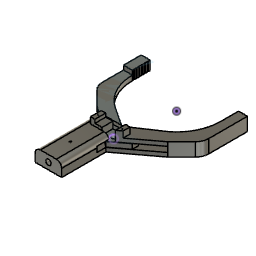
klo (Autodesk Fusion 360 design; units mm, degrees)
Autodesk Fusion 360 part; units mm, degrees
sketch "Sketch1" plane through (0, 0, 0) normal (0, 0, 1) x (1, 0, 0)
  circle A0 centre (0, 0) radius 50
  circle A1 centre (0, 0) radius 40 construction
  line L0 (45.8258, 20) -> (60, 20)
  line L1 (60, 20) -> (60, -30)
  line L2 (0, 0) -> (0, -40)
  line L3 (0, -60) -> (25.3846, -43.0769)
  line L4 (0, -80) -> (40, -50)
  line L5 (40, -50) -> (60, -30)
  line L6 (0, -80) -> (-30, -80)
  line L7 (-30, -60) -> (-30, -80)
  line L8 (0, -60) -> (-30, -60)
  dimension "d1" = 100
  constraint coincident A0.centre A1.centre
  constraint concentric A0 A1
  constraint perpendicular L0 L1
  constraint coincident A1 L2.end
  constraint coincident A0 L0.start
  constraint coincident A0 L3.end
  constraint horizontal L6
  constraint perpendicular L6 L7
  constraint perpendicular L7 L8
  measures "d1" diameter of A0
extrude "Extrude1" add sketch "Sketch1" along normal blind 15 contours A0 L0 L1 L3 L4 L5 L6 L7 L8 makes body 1
sketch "Sketch2" plane through (0, 0, 15) normal (0, 0, 1) x (-1, 0, 0)
  line L0 (-25.3846, 43.0769) -> (0, 60)
  line L1 (0, 60) -> (30, 60)
  line L2 (30, 60) -> (30, 80)
  line L3 (30, 80) -> (0, 80)
  line L4 (0, 80) -> (-40, 50)
  line L5 (-40, 50) -> (-60, 30)
  line L6 (-60, 30) -> (-60, -20)
  line L7 (-60, -20) -> (-45.8258, -20)
  arc A0 (-25.3846, 43.0769) -> (-45.8258, -20) centre (0, 0) ccw
  circle A1 centre (0, 70) radius 5
  dimension "d4" = 10
  measures "d4" diameter of A1
ref_plane "WorkPlane6" through (0, 0, 7.5) normal (0, 0, 1) x (1, 0, 0)
sketch "Sketch4" plane through (0, 0, 7.5) normal (0, 0, 1) x (1, 0, 0)
  circle A0 centre (0, 0) radius 50
  line L0 (60, 20) -> (45.8258, 20)
  line L1 (60, 20) -> (60, -30)
  line L2 (0, -80) -> (-30, -80)
  line L3 (-30, -80) -> (-30, -60)
  line L4 (-30, -60) -> (0, -60)
  line L5 (0, -60) -> (27.6385, -41.6667)
  line L6 (0, -80) -> (40, -50)
  line L7 (40, -50) -> (60, -30)
  line L8 (0, 2.5) -> (0, 20)
  line L9 (30, -60) -> (0, -60)
  line L10 (-60, 20) -> (-60, -30)
  circle A1 centre (0, 0) radius 50
  line L11 (0, -80) -> (30, -80)
  line L12 (-40, -50) -> (-60, -30)
  line L13 (0, -60) -> (-27.6385, -41.6667)
  line L14 (-60, 20) -> (-45.8258, 20)
  line L15 (0, -80) -> (-40, -50)
  line L16 (30, -80) -> (30, -60)
  constraint coincident A0.centre A1.centre
  constraint coincident A0 L0.end
  constraint horizontal L0
  constraint perpendicular L0 L1
  constraint perpendicular L1 L2
  constraint perpendicular L0 L3
  constraint perpendicular L3 L4
  constraint coincident A0 L5.end
  constraint tangent A0 L5
  constraint symmetric A0.centre L8 A1.centre
  constraint symmetric A0 L8 A1
  constraint symmetric L0.start L8 L10.start
  constraint symmetric L0.end L8 L14.end
  constraint symmetric L1.end L8 L10.end
  constraint symmetric L2.start L8 L6.start
  constraint symmetric L2.end L8 L11.end
  constraint symmetric L3.end L8 L9.start
  constraint symmetric L4.end L8 L5.start
  constraint symmetric L5.end L8 L13.end
  constraint symmetric L6.end L8 L12.start
extrude "Extrude1'" add sketch "Sketch4" along normal blind 2.75 and the other way blind 2.75 separate body contours A0 L4 L10 A1 L12 L13 L14 L15 | L4 L6 L9 L15 | L6 L9 L11 L16 makes body 2 in component "Component"
ref_plane "WorkPlane1" through (20, -65, 7.5) normal (0.6, -0.8, 0) x (0.8, 0.6, 0) in component "Component"
sketch "Sketch1 (2)" plane through (20, -65, 10) normal (0.6, -0.8, 0) x (0.8, 0.6, 0) in component "Component"
  line L0 (-25, 5) -> (11, 5)
  line L1 (11, 5) -> (11, -5)
  line L2 (11, -5) -> (-25, -5)
  line L3 (-25, -5) -> (-25, 5)
  constraint horizontal L0
  constraint perpendicular L0 L1
  constraint perpendicular L1 L2
extrude "Extrude2" cut sketch "Sketch1 (2)" along normal blind 22 bodies 2 in component "Component"
sketch "Sketch5" plane through (0, 0, 7.5) normal (0, 0, 1) x (1, 0, 0)
  line L0 (0, -60) -> (-30, -60)
  line L1 (-30, -60) -> (-30, -80)
  line L2 (-30, -80) -> (0, -80)
  line L3 (0, -80) -> (40, -50)
  line L4 (40, -50) -> (30, -40)
  line L5 (30, -40) -> (0, -60)
  constraint horizontal L0
  constraint perpendicular L0 L1
  constraint perpendicular L1 L2
extrude "Extrude3" cut sketch "Sketch5" along normal blind 3 and the other way blind 3 bodies 1
extrude "Extrude4" cut sketch "Sketch2" against normal blind 4.5 contours A1 bodies 1
extrude "Extrude3'" [no effect] in component "Component"
sketch "Sketch13" plane through (0, 0, 10.25) normal (0, 0, 1) x (-1, 0, 0)
  line L0 (0, 80) -> (-26.6667, 60)
  line L1 (-26.6667, 60) -> (0, 60)
  line L2 (0, 60) -> (27.6385, 41.6667)
  arc A0 (45.8258, -20) -> (27.6385, 41.6667) centre (0, 0) ccw
  line L3 (45.8258, -20) -> (60, -20)
  line L4 (60, -20) -> (60, 30)
  line L5 (60, 30) -> (40, 50)
  line L6 (40, 50) -> (0, 80)
  line L7 (0, 70) -> (0.2128, 70)
  line L8 (0, 66) -> (0, 74) construction
  circle A1 centre (0, 70) radius 3.5
  line L9 (-2.9142, 68.0616) -> (-13.1179, 63.9525)
  circle A2 centre (-13.1179, 63.9525) radius 2
  line L10 (-1.7875, 73.0091) -> (-14.1393, 65.672)
  line L11 (1.1273, 66.6865) -> (-12.4737, 62.0591)
  dimension "d58" = 7
  dimension "d61" = 11
  dimension "d62" = 4
  constraint vertical L8
  constraint coincident A1 L9.start
  constraint coincident L9.end A2.centre
  constraint coincident A1 L10.start
  constraint coincident A2 L10.end
  constraint tangent A2 L10
  constraint coincident A1 L11.start
  constraint coincident A2 L11.end
  constraint tangent A2 L11
  constraint tangent A1 L11
  constraint tangent A1 L10
  measures "d58" diameter of A1
  measures "d61" distance of L9.start L9.end
  measures "d62" diameter of A2
sketch "Sketch14" plane through (0, 0, 0) normal (0, 0, -1) x (1, 0, 0)
  line L0 (0, 60) -> (25.3846, 43.0769)
  arc A0 (45.8258, -20) -> (25.3846, 43.0769) centre (0, 0) ccw
  line L1 (45.8258, -20) -> (60, -20)
  line L2 (60, -20) -> (60, 30)
  line L3 (60, 30) -> (40, 50)
  line L4 (40, 50) -> (0, 80)
  line L5 (0, 80) -> (-30, 80)
  line L6 (-30, 80) -> (-30, 60)
  line L7 (-30, 60) -> (0, 60)
  circle A1 centre (0, 70) radius 5
sketch "Sketch6" plane through (0, -80, 0) normal (0, -1, 0) x (1, 0, 0)
  line L0 (0, 10.5) -> (0, 15)
  line L1 (-30, 15) -> (-30, 10.5)
  line L2 (-30, 15) -> (0, 15)
  line L3 (0, 15) -> (0, 0)
  line L4 (0, 0) -> (-30, 0)
  line L5 (-30, 0) -> (-30, 15)
  line L6 (-30, 10.5) -> (0, 10.5)
  line L7 (0, 15) -> (-30, 15)
  constraint horizontal L2
  constraint vertical L3
  constraint horizontal L4
  constraint vertical L5
  constraint coincident L3.end L4.start
  constraint coincident L1.start L2.start
sketch "Sketch7" plane through (0, 0, 10.25) normal (0, 0, 1) x (-1, 0, 0)
  line L0 (0, 80) -> (-26.6667, 60)
  line L1 (-26.6667, 60) -> (0, 60)
  line L2 (0, 60) -> (27.6385, 41.6667)
  arc A0 (45.8258, -20) -> (27.6385, 41.6667) centre (0, 0) ccw
  line L3 (45.8258, -20) -> (60, -20)
  line L4 (60, -20) -> (60, 30)
  line L5 (60, 30) -> (40, 50)
  line L6 (40, 50) -> (0, 80)
  line L7 (-10, 60) -> (-10, 72.5)
  line L8 (-26.6667, 60) -> (-10, 60)
  line L9 (-10, 72.5) -> (-26.6667, 60)
  constraint coincident L1 L7.start
  constraint coincident L0 L7.end
  constraint perpendicular L1 L7
  constraint coincident L0.end L1.start
  constraint perpendicular L7 L8
  constraint parallel L0 L9
extrude "Extrude4'" cut sketch "Sketch7" against normal blind 30 contours L0 L1 L7 L8 L9 bodies 2 in component "Component"
sketch "Sketch8" plane through (0, -80, 0) normal (0, -1, 0) x (1, 0, 0)
  line L0 (0, 10.5) -> (0, 15)
  line L1 (-30, 15) -> (-30, 10.5)
  line L2 (-30, 15) -> (0, 15)
  line L3 (0, 15) -> (0, 10.5)
  line L4 (0, 10.5) -> (-30, 10.5)
  line L5 (-30, 10.5) -> (-30, 15)
  line L6 (-30, 4.5) -> (0, 4.5)
  line L7 (0, 4.5) -> (0, 0)
  line L8 (0, 0) -> (-30, 0)
  line L9 (-30, 0) -> (-30, 4.5)
  line L10 (-30, 10.5) -> (0, 10.5)
  line L11 (0, 15) -> (-30, 15)
  constraint horizontal L2
  constraint vertical L3
  constraint horizontal L4
  constraint vertical L5
  constraint coincident L0.start L3.end
  constraint coincident L1.start L2.start
  constraint horizontal L6
  constraint vertical L7
  constraint horizontal L8
  constraint vertical L9
  constraint coincident L7.end L8.start
extrude "Extrude6" add sketch "Sketch8" along normal blind 10 bodies 1
sketch "Sketch9" plane through (0, -90, 0) normal (0, -1, 0) x (1, 0, 0)
  line L0 (-30, 10.5) -> (0, 10.5)
  line L1 (0, 10.5) -> (0, 15)
  line L2 (0, 15) -> (-30, 15)
  line L3 (-30, 15) -> (-30, 10.5)
  line L4 (-30, 15) -> (0, 15)
  line L5 (0, 15) -> (0, 0)
  line L6 (0, 0) -> (-30, 0)
  line L7 (-30, 0) -> (-30, 15)
  constraint horizontal L4
  constraint vertical L5
  constraint horizontal L6
  constraint vertical L7
  constraint coincident L5.end L6.start
  constraint coincident L2.end L3.start
extrude "Extrude7" add sketch "Sketch9" along normal blind 40 bodies 1
ref_plane "WorkPlane7" through (-15, -131, 7.5) normal (0, -1, 0) x (0, 0, -1)
sketch "Sketch10" plane through (-15, -131, 10) normal (0, -1, 0) x (1, 0, 0)
  line L0 (-15, 10) -> (15, 10)
  line L1 (15, 10) -> (15, -10)
  line L2 (15, -10) -> (-15, -10)
  line L3 (-15, -10) -> (-15, 10)
  constraint horizontal L0
  constraint vertical L1
  constraint horizontal L2
  constraint vertical L3
copy_body "Body->Comp3" bodies 1 removing the originals makes body 3 in component "Component'"
sketch "Sketch12" plane through (0, -130, 0) normal (0, -1, 0) x (1, 0, 0)
  line L0 (-30, 0) -> (0, 0)
  line L1 (0, 0) -> (0, 15)
  line L2 (0, 15) -> (-30, 15)
  line L3 (-30, 15) -> (-30, 0)
  circle A0 centre (-15, 7.5) radius 3
  dimension "d50" = 6
  measures "d50" diameter of A0
extrude "Extrude1''" cut sketch "Sketch12" against normal blind 40 contours A0 bodies 3 in component "Component'"
sketch "Sketch15" plane through (10, 0, 0) normal (1, 0, 0) x (0, 1, 0)
  line L0 (-72.5, 4.75) -> (-60, 4.75)
  line L1 (-60, 4.75) -> (-60, 10.25)
  line L2 (-60, 10.25) -> (-72.5, 10.25)
  line L3 (-72.5, 10.25) -> (-72.5, 5)
  line L4 (-72.5, 10.25) -> (-60, 10.25)
  line L5 (-60, 10.25) -> (-60, 4.75)
  line L6 (-60, 4.75) -> (-72.5, 4.75)
  line L7 (-72.5, 4.75) -> (-72.5, 10.25)
  line L8 (-72.5, 5) -> (-72.5, 4.75)
  constraint horizontal L4
  constraint vertical L5
  constraint horizontal L6
  constraint vertical L7
  constraint coincident L0.end L1.start
  constraint coincident L2.end L3.start
extrude "Extrude6'" add sketch "Sketch15" along normal blind 7 bodies 2 in component "Component"
extrude "Extrude7'" cut sketch "Sketch13" against normal blind 5.5 contours A1 | A1 L9 A2 L10 | A1 L9 A2 L11 | A2 bodies 2 in component "Component"
ref_plane "WorkPlane8" through (20, -65, 12.75) normal (0.6, -0.8, 0) x (0.8, 0.6, 0)
sketch "Sketch16" plane through (20, -65, 12.75) normal (0.6, -0.8, 0) x (0.8, 0.6, 0)
  line L0 (-12.8308, -2.59) -> (4, -2.59)
  line L1 (4, -2.59) -> (4, -8)
  line L2 (4, -8) -> (-12.8308, -8)
  line L3 (-12.8308, -8) -> (-12.8308, -2.59)
  constraint horizontal L0
  constraint vertical L1
  constraint horizontal L2
  constraint vertical L3
extrude "Extrude8" cut sketch "Sketch16" along normal blind 20 bodies 2 makes body 4 at (26.6222, -64.7556, 5) in component "Component"
sketch "Sketch17" plane through (0, 0, 15) normal (0, 0, 1) x (-1, 0, 0)
  circle A0 centre (0, 70) radius 5
  line L0 (-25.3846, 43.0769) -> (0, 60)
  line L1 (0, 60) -> (30, 60)
  line L2 (30, 60) -> (30, 130)
  line L3 (30, 130) -> (0, 130)
  line L4 (0, 130) -> (0, 80)
  line L5 (0, 80) -> (-40, 50)
  line L6 (-40, 50) -> (-60, 30)
  line L7 (-60, 30) -> (-60, -20)
  line L8 (-60, -20) -> (-45.8258, -20)
  arc A1 (-25.3846, 43.0769) -> (-45.8258, -20) centre (0, 0) ccw
  circle A2 centre (0, 70) radius 6.15
  line L9 (-6.15, 70) -> (-6.15, 63.85)
  line L10 (-6.15, 63.85) -> (8.25, 63.85)
  line L11 (8.25, 63.85) -> (8.25, 76.15)
  line L12 (8.25, 76.15) -> (-6.15, 76.15)
  line L13 (-6.15, 76.15) -> (-6.15, 63.85)
  dimension "d70" = 12.3
  dimension "d74" = 12.3
  dimension "d75" = 14.4
  constraint concentric A0 A2
  constraint coincident A2 L9.start
  constraint tangent A2 L9
  constraint vertical L9
  constraint horizontal L10
  constraint vertical L11
  constraint horizontal L12
  constraint vertical L13
  constraint tangent A2 L10
  measures "d70" diameter of A2
  measures "d74" distance of L10.end L11.end
  measures "d75" distance of L9.end L10.end
sketch "Sketch18" plane through (0, 0, 15) normal (0, 0, 1) x (-1, 0, 0)
  line L0 (15, 130) -> (15, 105)
  circle A0 centre (15, 105) radius 1
  dimension "d71" = 2
  constraint vertical L0
  constraint coincident L0.end A0.centre
  measures "d71" diameter of A0
extrude "Extrude2'" cut sketch "Sketch18" against normal blind 35 bodies 3 in component "Component'"
extrude "Extrude3''" cut sketch "Sketch17" against normal blind 4.5 contours L5 A2 L12 L13 | A2 | A2 L9 L10 L13 | A2 L10 L11 L12 bodies 3 in component "Component'"
sketch "Sketch19" plane through (0, 0, 15) normal (0, 0, 1) x (-1, 0, 0)
  line L0 (-5.1333, 76.15) -> (8.25, 76.15)
  line L1 (8.25, 76.15) -> (8.25, 63.85)
  line L2 (8.25, 63.85) -> (-6.15, 63.85)
  line L3 (-6.15, 63.85) -> (-6.15, 75.3875)
  line L4 (-6.15, 75.3875) -> (-40, 50)
  line L5 (-40, 50) -> (-60, 30)
  line L6 (-60, 30) -> (-60, -20)
  line L7 (-60, -20) -> (-45.8258, -20)
  arc A0 (-25.3846, 43.0769) -> (-45.8258, -20) centre (0, 0) ccw
  line L8 (-25.3846, 43.0769) -> (0, 60)
  line L9 (0, 60) -> (30, 60)
  line L10 (30, 60) -> (30, 130)
  line L11 (30, 130) -> (0, 130)
  line L12 (0, 130) -> (0, 80)
  line L13 (0, 80) -> (-5.1333, 76.15)
  circle A1 centre (15, 105) radius 1
  line L14 (8.25, 63.85) -> (16.25, 63.85)
  line L15 (16.25, 63.85) -> (16.25, 76.15)
  line L16 (16.25, 76.15) -> (8.25, 76.15)
  line L17 (8.25, 76.15) -> (8.25, 63.85)
  line L18 (16.25, 63.85) -> (21.25, 63.85)
  line L19 (21.25, 63.85) -> (21.25, 76.15)
  line L20 (21.25, 76.15) -> (16.25, 76.15)
  line L21 (16.25, 76.15) -> (16.25, 63.85)
  line L22 (-6.15, 63.85) -> (-11.15, 63.85)
  line L23 (-11.15, 63.85) -> (-11.15, 76.15)
  line L24 (-11.15, 76.15) -> (-6.15, 76.15)
  line L25 (-6.15, 76.15) -> (-6.15, 63.85)
  dimension "d78" = 8
  dimension "d79" = 5
  dimension "d80" = 5
  constraint horizontal L14
  constraint vertical L15
  constraint horizontal L16
  constraint vertical L17
  constraint coincident L1.end L2.start
  constraint horizontal L18
  constraint vertical L19
  constraint horizontal L20
  constraint vertical L21
  constraint horizontal L22
  constraint vertical L23
  constraint horizontal L24
  constraint vertical L25
  constraint coincident L2.end L3.start
  measures "d78" distance of L15.end L0.end
  measures "d79" distance of L19.end L15.end
  measures "d80" distance of L2.end L22.end
extrude "Extrude4''" add sketch "Sketch19" along normal blind 7 contours L15 L18 L19 L20 L21 | L3 L4 L22 L23 L25 bodies 3 in component "Component'"
sketch "Sketch20" plane through (38.4, -51.2, 0) normal (0.6, -0.8, 0) x (0.8, 0.6, 0)
  line L0 (-40.3125, 22) -> (-40.3125, 10.5)
  line L1 (-40.3125, 10.5) -> (2, 10.5)
  line L2 (2, 10.5) -> (2, 15)
  line L3 (2, 15) -> (-34.0625, 15)
  line L4 (-34.0625, 15) -> (-34.0625, 22)
  line L5 (-34.0625, 22) -> (-40.3125, 22)
  line L6 (-48, 15) -> (2, 15)
  line L7 (2, 15) -> (2, 0)
  line L8 (2, 0) -> (-48, 0)
  line L9 (-48, 0) -> (-48, 15)
  constraint horizontal L6
  constraint vertical L7
  constraint horizontal L8
  constraint vertical L9
extrude "Extrude9" cut sketch "Sketch20" along normal blind 14 contours L0 L1 L2 L3 L6 L7 | L0 L1 L6 L7 L8 L9 bodies 2 4 in component "Component"
sketch "Sketch21" plane through (0, 0, 7.5) normal (0, 0, 1) x (1, 0, 0)
  circle A0 centre (0, 0) radius 50
  line L0 (-60, 20) -> (-45.8258, 20)
  line L1 (-60, 20) -> (-60, 0)
  line L2 (-60, 0) -> (-50, 0)
  constraint coincident A0.centre origin
  constraint coincident A0 L0.end
  constraint horizontal L0
  constraint perpendicular L0 L1
  constraint coincident A0 L2.end
  constraint perpendicular L1 L2
extrude "Extrude10" add sketch "Sketch21" along normal blind 7.5 contours A0 L0 L1 L2 bodies 2 4 in component "Component"
sketch "Sketch22" plane through (0, 0, 4.5) normal (0, 0, 1) x (-1, 0, 0)
  arc A0 (-25.3846, 43.0769) -> (-30, 40) centre (0, 0) ccw
  line L0 (-25.3846, 43.0769) -> (0, 60)
  line L1 (0, 60) -> (30, 60)
  line L2 (30, 60) -> (30, 90)
  line L3 (30, 90) -> (15, 90)
  line L4 (15, 90) -> (0, 90)
  line L5 (0, 90) -> (0, 80)
  line L6 (0, 80) -> (-40, 50)
  line L7 (-40, 50) -> (-30, 40)
  circle A1 centre (0, 70) radius 3.5
  dimension "d89" = 7
  measures "d89" diameter of A1
extrude "Extrude5" add sketch "Sketch22" along normal blind 0.5 contours A1 bodies 3 in component "Component'"
sketch "Sketch23" plane through (0, 0, 10.25) normal (0, 0, 1) x (-1, 0, 0)
  line L0 (50, 0) -> (60, 0)
  line L1 (60, 0) -> (60, 30)
  line L2 (60, 30) -> (40, 50)
  line L3 (40, 50) -> (0, 80)
  line L4 (0, 80) -> (-17, 67.25)
  line L5 (-17, 67.25) -> (-17, 60)
  line L6 (-17, 60) -> (0, 60)
  line L7 (0, 60) -> (27.6385, 41.6667)
  arc A0 (50, 0) -> (27.6385, 41.6667) centre (0, 0) ccw
  arc A1 (-14.1393, 65.672) -> (-12.4737, 62.0591) centre (-13.1179, 63.9525) ccw
  line L8 (-14.1393, 65.672) -> (-1.7875, 73.0091)
  arc A2 (1.1273, 66.6865) -> (-1.7875, 73.0091) centre (0, 70) ccw
  line L9 (1.1273, 66.6865) -> (-12.4737, 62.0591)
sketch "Sketch24" plane through (0, 0, 22) normal (0, 0, 1) x (-1, 0, 0)
  line L0 (16.25, 76.15) -> (16.25, 63.85)
  line L1 (16.25, 63.85) -> (21.25, 63.85)
  line L2 (21.25, 63.85) -> (21.25, 76.15)
  line L3 (21.25, 76.15) -> (16.25, 76.15)
  circle A0 centre (18.75, 70) radius 0.5
  circle A1 centre (-8.65, 70) radius 0.5
  line L4 (-11.15, 63.85) -> (-6.15, 63.85)
  line L5 (-8.65, 63.85) -> (-8.65, 72)
  dimension "d94" = 1
  dimension "d95" = 1
  constraint midpoint L4 L5.start
  constraint perpendicular L4 L5
  constraint coincident A1.centre L5
  measures "d94" diameter of A0
  measures "d95" diameter of A1
sketch "Sketch25" plane through (0, 0, 15) normal (0, 0, 1) x (-1, 0, 0)
  line L0 (-11.15, 63.85) -> (-11.15, 71.6375)
  line L1 (-11.15, 71.6375) -> (-40, 50)
  line L2 (-40, 50) -> (-60, 30)
  line L3 (-60, 30) -> (-60, -20)
  line L4 (-60, -20) -> (-45.8258, -20)
  arc A0 (-25.3846, 43.0769) -> (-45.8258, -20) centre (0, 0) ccw
  line L5 (-25.3846, 43.0769) -> (0, 60)
  line L6 (0, 60) -> (30, 60)
  line L7 (30, 60) -> (30, 130)
  line L8 (30, 130) -> (0, 130)
  line L9 (0, 130) -> (0, 80)
  line L10 (0, 80) -> (-5.1333, 76.15)
  line L11 (-5.1333, 76.15) -> (8.25, 76.15)
  line L12 (8.25, 76.15) -> (8.25, 63.85)
  line L13 (8.25, 63.85) -> (-6.15, 63.85)
  line L14 (-6.15, 63.85) -> (-11.15, 63.85)
  line L15 (16.25, 76.15) -> (21.25, 76.15)
  line L16 (21.25, 76.15) -> (21.25, 63.85)
  line L17 (21.25, 63.85) -> (16.25, 63.85)
  line L18 (16.25, 63.85) -> (16.25, 76.15)
  circle A1 centre (15, 105) radius 1
  line L19 (16.25, 63.85) -> (8.25, 63.85)
  line L20 (8.25, 63.85) -> (8.25, 76.15)
  line L21 (8.25, 76.15) -> (16.25, 76.15)
  line L22 (16.25, 76.15) -> (16.25, 63.85)
  constraint horizontal L19
  constraint vertical L20
  constraint horizontal L21
  constraint vertical L22
  constraint coincident L11.end L12.start
  constraint coincident L17.end L18.start
extrude "Extrude6''" add sketch "Sketch25" along normal blind 3 contours L12 L18 L19 L20 L21 L22 bodies 3 in component "Component'"
extrude "Extrude7''" cut sketch "Sketch24" against normal blind 0.5 contours A0 | A1 L5 | A1 L5 bodies 3 in component "Component'"
fillet "Fillet1" radius 6 2 edges at (0, -105, 15) (-30, -95, 15) on bodies 3 in component "Component'"
sketch "Sketch26" plane through (0, 0, 15) normal (0, 0, 1) x (-1, 0, 0)
  line L0 (60, -20) -> (60, 0)
  line L1 (60, 0) -> (50, 0)
  arc A0 (45.8258, -20) -> (50, 0) centre (0, 0) ccw
  line L2 (45.8258, -20) -> (60, -20)
ref_plane "WorkPlane9" through (-50, 0, 0) normal (1, 0, 0) x (0, 1, 0)
sketch "Sketch27" plane through (-50, 0, 0) normal (1, 0, 0) x (0, 1, 0)
  line L0 (0, 15) -> (22, 15)
  line L1 (22, 15) -> (22, -1)
  line L2 (22, -1) -> (0, -1)
  line L3 (0, -1) -> (0, 15)
  constraint horizontal L0
  constraint vertical L1
  constraint horizontal L2
  constraint vertical L3
extrude "Extrude11" cut sketch "Sketch27" along normal blind 100 bodies 2 in component "Component"
extrude "Extrude8'" cut sketch "Sketch27" along normal blind 100 bodies 3 in component "Component'"
sketch "Sketch28" plane through (0, 0, 0) normal (0, 0, 1) x (1, 0, 0)
fillet "Fillet2" radius 15 1 edges at (60, -30, 7.5) on bodies 3 in component "Component'"
fillet "Fillet1'" radius 15 1 edges at (-60, -30, 7.5) on bodies 2 in component "Component"
sketch "Sketch29" plane through (-50, 0, 0) normal (1, 0, 0) x (0, 1, 0)
  line L0 (20, 4.75) -> (20, 15)
  line L1 (20, 15) -> (0, 15)
  line L2 (0, 15) -> (0, 10.25)
  line L3 (0, 10.25) -> (0, 4.75)
  line L4 (1, 0) -> (2.0404, 0)
  line L5 (2.0404, 0) -> (2.0404, 15)
  line L6 (2.0404, 15) -> (1, 15)
  line L7 (1, 15) -> (1, 0)
  line L8 (5.2404, 0) -> (5.2404, 15)
  line L9 (4.2, 15) -> (4.2, 0)
  line L10 (5.2404, 15) -> (4.2, 15)
  line L11 (4.2, 0) -> (5.2404, 0)
  line L12 (8.4404, 0) -> (8.4404, 15)
  line L13 (7.4, 15) -> (7.4, 0)
  line L14 (8.4404, 15) -> (7.4, 15)
  line L15 (7.4, 0) -> (8.4404, 0)
  line L16 (11.6404, 0) -> (11.6404, 15)
  line L17 (10.6, 15) -> (10.6, 0)
  line L18 (11.6404, 15) -> (10.6, 15)
  line L19 (10.6, 0) -> (11.6404, 0)
  line L20 (14.8404, 0) -> (14.8404, 15)
  line L21 (13.8, 15) -> (13.8, 0)
  line L22 (14.8404, 15) -> (13.8, 15)
  line L23 (13.8, 0) -> (14.8404, 0)
  line L24 (18.0404, 0) -> (18.0404, 15)
  line L25 (17, 15) -> (17, 0)
  line L26 (18.0404, 15) -> (17, 15)
  line L27 (17, 0) -> (18.0404, 0)
  line L28 (0, 4.75) -> (20, 4.75)
  dimension "d111" = 16
  dimension "d112" = 0
  constraint horizontal L4
  constraint vertical L5
  constraint horizontal L6
  constraint vertical L7
  constraint coincident L1 L5.end
extrude "Extrude12" cut sketch "Sketch29" against normal blind 0.25 contours L1 L24 L25 L26 L28 | L24 L25 L27 L28 | L1 L20 L21 L22 L28 | L20 L21 L23 L28 | L1 L16 L17 L18 L28 | L16 L17 L19 L28 | L1 L12 L13 L14 L28 | L12 L13 L15 L28 | L1 L8 L9 L10 L28 | L8 L9 L11 L28 | L1 L5 L6 L7 L28 | L4 L5 L7 L28 bodies 2 in component "Component"
component "Component" placed x (1, 0, 0) y (0, 1, 0) z (0, 0, 1) at (0, 0, 0)
component "Component'" placed x (1, 0, 0) y (0, 1, 0) z (0, 0, 1) at (0, 0, 0)
